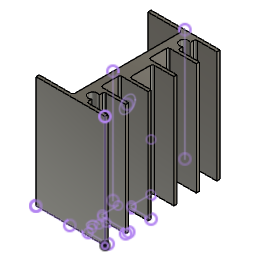
motor_driver_final (Autodesk Fusion 360 archive; units mm, degrees)
design "heat_sink"
Autodesk Fusion 360 part; units mm, degrees
sketch "Sketch1" plane through (0, 0, 0) normal (1, 0, 0) x (0, 1, 0)
  line L0 (0, 0) -> (25.696, 0)
  line L1 (25.696, 0) -> (25.696, 25)
  line L2 (25.696, 25) -> (0, 25)
  line L3 (0, 25) -> (0, 0)
  dimension "d1" = 25.696
  dimension "d2" = 25
  constraint horizontal L0
  constraint vertical L1
  constraint horizontal L2
  constraint vertical L3
  constraint coincident L0.start L3.end
  measures "d1" distance of L0.start L0.end
  measures "d2" distance of L0.start L2.end
extrude "Extrude1" add sketch "Sketch1" along normal blind 3.046
sketch "Sketch4" plane through (3.046, 0, 0) normal (1, 0, 0) x (0, 1, 0)
  line L0 (0, 25) -> (0, 0)
  line L1 (0, 0) -> (25.696, 0)
  line L2 (25.696, 0) -> (25.696, 25)
  line L3 (25.696, 25) -> (0, 25)
  line L4 (0, 0) -> (0.696, 0)
  line L5 (0.696, 0) -> (0.696, 25)
  line L6 (0.696, 25) -> (0, 25)
  line L7 (0, 25) -> (0, 0)
  line L8 (12.848, 25) -> (12.848, 0) construction
  line L9 (25.696, 25) -> (25.696, 0)
  line L10 (25, 0) -> (25, 25)
  dimension "d15" = 0.696
  dimension "d16" = 25
  constraint horizontal L4
  constraint vertical L5
  constraint horizontal L6
  constraint vertical L7
  constraint coincident L0.end L1.start
  constraint midpoint L3 L8.start
  constraint midpoint L1 L8.end
  constraint symmetric L0.end L8 L1.end
  constraint symmetric L4.end L8 L10.start
  constraint symmetric L5.end L8 L10.end
  constraint symmetric L0.start L8 L2.end
  measures "d15" distance of L0.end L4.end
  measures "d16" distance of L0.end L0.start
extrude "Extrude3" add sketch "Sketch4" along normal blind 4.8 and the other way blind 10.6 contours L0 L1 L3 L4 L5 L6 L7 | L1 L2 L3 L9 L10
sketch "Sketch5" plane through (3.046, 0, 0) normal (1, 0, 0) x (0, 1, 0)
  line L0 (25, 0) -> (25, 25)
  line L1 (25, 25) -> (0.696, 25)
  line L2 (0.696, 25) -> (0.696, 0)
  line L3 (0.696, 0) -> (25, 0)
  line L4 (4.63, 25) -> (4.63, 0)
  line L5 (5.294, 25) -> (5.294, 0)
  line L6 (9.63, 25) -> (9.63, 0)
  line L7 (10.294, 25) -> (10.294, 0)
  line L8 (12.848, 25) -> (12.848, 0) construction
  line L9 (21.066, 25) -> (21.066, 0)
  line L10 (20.402, 25) -> (20.402, 0)
  line L11 (16.066, 25) -> (16.066, 0)
  line L12 (15.402, 25) -> (15.402, 0)
  dimension "d21" = -3.934
  dimension "d22" = -4.598
  dimension "d23" = -8.934
  dimension "d24" = -9.598
  constraint midpoint L1 L8.start
  constraint midpoint L3 L8.end
  constraint symmetric L4.start L8 L9.start
  constraint symmetric L4.end L8 L9.end
  constraint symmetric L5.start L8 L10.start
  constraint symmetric L5.end L8 L10.end
  constraint symmetric L6.start L8 L11.start
  constraint symmetric L6.end L8 L11.end
  constraint symmetric L7.start L8 L12.start
  constraint symmetric L7.end L8 L12.end
extrude "Extrude4" add sketch "Sketch5" along normal blind 4.8 contours L1 L3 L9 L10 | L1 L3 L11 L12 | L1 L3 L6 L7 | L1 L3 L4 L5
sketch "Sketch6" plane through (0, 0, 0) normal (0, 0, 1) x (1, 0, 0)
  circle A0 centre (2.4572, 2.6766) radius 1
  line L0 (0, 0) -> (0, 25.696)
  line L1 (0, 12.848) -> (3.046, 12.848) construction
  circle A1 centre (2.4572, 23.0194) radius 1
  dimension "d27" = 2
  dimension "d28" = 25.696
  dimension "d29" = 3.046
  constraint coincident L0.start origin
  constraint vertical L0
  constraint midpoint L0 L1.start
  constraint perpendicular L0 L1
  constraint symmetric A0 L1 A1
  measures "d27" diameter of A0
  measures "d28" distance of L0.start L0.end
  measures "d29" distance of L1.start L1.end
extrude "Extrude5" cut sketch "Sketch6" along normal blind 25
sketch "Sketch7" plane through (0, 0, 0) normal (1, 0, 0) x (0, 1, 0)
sketch "Sketch8" plane through (3.046, 0, 0) normal (1, 0, 0) x (0, 1, 0)
  line L0 (15.402, 0) -> (15.402, 25)
  line L1 (15.402, 25) -> (10.294, 25)
  line L2 (10.294, 25) -> (10.294, 0)
  line L3 (10.294, 0) -> (15.402, 0)
  line L4 (12.848, 0) -> (12.848, 17) construction
  circle A0 centre (12.848, 17) radius 1.75
  dimension "d32" = 3.5
  constraint midpoint L3 L4.start
  constraint perpendicular L3 L4
  constraint coincident L4.end A0.centre
  measures "d32" diameter of A0
extrude "Extrude6" cut sketch "Sketch8" against normal blind 3.046 contours A0
sketch "Sketch9" plane through (0, 0, 0) normal (0, 0, 1) x (1, 0, 0)
sketch "Sketch10" plane through (0, 0, 0) normal (1, 0, 0) x (0, 1, 0)
extrude "Extrude7" cut 1 faces at (3.046, 8.1847, 8.3333) along direction (-1, 0, 0) blind 1.5
sketch "Sketch11" plane through (0, 0, 0) normal (1, 0, 0) x (0, 1, 0)
extrude "Extrude8" cut 1 faces at (3.046, 17.5113, 8.3333) along direction (-1, 0, 0) blind 1.5
fillet "Fillet1" radius 0.4 10 edges at (3.046, 0.696, 12.5) (3.046, 4.63, 12.5) (1.546, 9.63, 12.5) (3.046, 15.402, 12.5) (1.546, 20.402, 12.5) (3.046, 25, 12.5) (1.546, 5.294, 12.5) (3.046, 10.294, 12.5) (1.546, 16.066, 12.5) (3.046, 21.066, 12.5)
fillet "Fillet2" radius 0.4 2 edges at (0, 25, 12.5) (0, 0.696, 12.5)
sketch "Sketch12" plane through (0, 0, 0) normal (1, 0, 0) x (0, 1, 0)
  line L0 (25.696, 25) -> (25.696, 0)
  circle A0 centre (12.848, 17) radius 1.75
  dimension "d45" = 25
  dimension "d46" = 25.696
  dimension "d47" = 3.5
  measures "d45" distance of L0.start L0.end
  measures "d46" distance of L0.end origin
  measures "d47" diameter of A0
sketch "Sketch13" plane through (0, 0, 0) normal (0, 1, 0) x (1, 0, 0)
  line L0 (7.846, -25) -> (7.846, 0)
  line L1 (-7.554, 0) -> (7.846, 0)
  dimension "d48" = 25
  dimension "d49" = 15.4
  measures "d48" distance of L0.start L0.end
  measures "d49" distance of L0.end L1.start
sketch "Sketch14" plane through (0, 0, 0) normal (0, 0, 1) x (1, 0, 0)
  arc A0 (3.046, 3.4849) -> (3.046, 1.8683) centre (2.4572, 2.6766) ccw
  line L0 (3.446, 4.63) -> (7.846, 4.63)
  line L1 (7.846, 5.294) -> (1.946, 5.294)
  line L2 (1.546, 5.694) -> (1.546, 9.23)
  line L3 (3.046, 15.002) -> (3.046, 10.694)
  line L4 (3.446, 10.294) -> (7.846, 10.294)
  line L5 (3.446, 0.696) -> (7.846, 0.696)
  point P0 (-7.554, 0)
  point P1 (-7.554, 25.696)
  dimension "d50" = 25.696
  dimension "d51" = 1
  dimension "d53" = 5.9
  dimension "d54" = 3.536
  dimension "d55" = 4.308
  dimension "d56" = 4.4
  dimension "d57" = 4.4
  measures "d50" distance of P0 P1
  measures "d51" radius of A0
  measures "d53" distance of L1.start L1.end
  measures "d54" distance of L2.start L2.end
  measures "d55" distance of L3.start L3.end
  measures "d56" distance of L4.start L4.end
  measures "d57" distance of L5.start L5.end
sketch "Sketch15" plane through (0, 0, 0) normal (1, 0, 0) x (0, 1, 0)
  line L0 (9.63, 25) -> (9.63, 0)
  dimension "d58" = 25
  measures "d58" distance of L0.start L0.end
equation "d6 = -0.696 mm - 3.934 mm"
equation "d7 = -0.696 mm - 3.934 mm - 0.664 mm"
equation "d8 = -0.696 mm - 3.934 mm - 0.664 mm - 4.336 mm"
equation "d9 = -0.696 mm - 3.934 mm - 0.664 mm - 4.336 mm - 0.664 mm"
equation "d19 = 3.046 mm + 7.554 mm"
equation "d22 = -3.934 mm - 0.664 mm"
equation "d23 = -3.934 mm - 0.664 mm - 4.336 mm"
equation "d24 = -3.934 mm - 0.664 mm - 4.336 mm - 0.664 mm"
